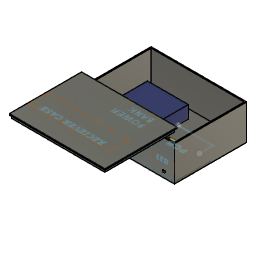
RECIEVER CASE (Autodesk Fusion 360 design; units mm, degrees)
part number: 2025-07-09-13-49-54-676
Autodesk Fusion 360 part; units mm, degrees
sketch "Sketch1" plane through (0, 0, 0) normal (0, 0, 1) x (1, 0, 0)
  line L0 (82, -62) -> (-82, -62)
  line L1 (-82, -62) -> (-82, 62)
  line L2 (-82, 62) -> (82, 62)
  line L3 (82, 62) -> (82, -62)
  line L4 (82, -62) -> (-82, 62) construction
  line L5 (-82, -62) -> (82, 62) construction
  dimension "d1" = 164
  dimension "d2" = 124
  constraint horizontal L0
  constraint perpendicular L0 L1
  constraint parallel L0 L2
  constraint parallel L1 L3
  constraint coincident L4 origin
  constraint coincident L5 origin
  measures "d1" distance of L1.end L2.end
  measures "d2" distance of L0.end L1.end
extrude "Extrude1" add sketch "Sketch1" along normal blind 60 makes body 1
shell "Shell1" thickness 2 removed faces 1 at (27.3333, -20.6667, 60) on bodies 1
sketch "Sketch2" plane through (0, 0, 0) normal (0, 0, 1) x (1, 0, 0)
  line L0 (82, -62) -> (-82, -62)
  line L1 (-82, -62) -> (-82, 62)
  line L2 (-82, 62) -> (82, 62)
  line L3 (82, 62) -> (82, -62)
  line L4 (82, -62) -> (-82, 62) construction
  line L5 (-82, -62) -> (82, 62) construction
  dimension "d6" = 164
  dimension "d7" = 124
  constraint horizontal L0
  constraint perpendicular L0 L1
  constraint parallel L0 L2
  constraint parallel L1 L3
  constraint coincident L4 origin
  constraint coincident L5 origin
  measures "d6" distance of L1.end L2.end
  measures "d7" distance of L0.end L1.end
extrude "Extrude2" add sketch "Sketch2" along normal blind 7 separate body makes body 2
move_body "Move1" bodies 2 to x (1, 0, 0) y (0, 1, 0) z (0, 0, 1) at (0, 0, 60)
sketch "Sketch3" plane through (0, 0, 67) normal (0, 0, 1) x (-1, 0, 0)
  line L0 (-82, -62) -> (82, -62)
  line L1 (82, -62) -> (82, 62)
  line L2 (82, 62) -> (-82, 62)
  line L3 (-82, 62) -> (-82, -62)
  line L4 (80, -60) -> (80, 60)
  line L5 (80, 60) -> (-80, 60)
  line L6 (-80, 60) -> (-80, -60)
  line L7 (-80, -60) -> (80, -60)
  dimension "d10" = -2
extrude "Extrude3" cut sketch "Sketch3" against normal blind 5 bodies 2
move_body "Move2" bodies 2 to x (-1, 0, 0) y (0, 1, 0) z (0, 0, -1) at (0, 0, 122)
sketch "Sketch4" plane through (0, -62, 0) normal (0, -1, 0) x (1, 0, 0)
  line L0 (-82, 0) -> (82, 0)
  line L1 (82, 0) -> (82, 60)
  line L2 (82, 60) -> (-82, 60)
  line L3 (-82, 60) -> (-82, 0)
  circle A0 centre (63.8545, 9.878) radius 2.5
  dimension "d13" = 5
  measures "d13" diameter of A0
extrude "Extrude4" cut sketch "Sketch4" against normal blind 5 contours A0 bodies 1
move_body "Move3" bodies 2 to x (1, 0, 0) y (0, 1, 0) z (0, 0, 1) at (0, 0, 30)
move_body "Move4" bodies 2 to x (1, 0, 0) y (0, 1, 0) z (0, 0, 1) at (0.6658, 0, -29.0981)
move_body "Move5" bodies 2 to x (1, 0, 0) y (0, 1, 0) z (0, 0, 1) at (0, 0, 50)
move_body "Move6" bodies 2 to x (1, 0, 0) y (0, 1, 0) z (0, 0, 1) at (0, 120, 0)
other "Base Mesh Feature1"
other "Scale1"
other "Modify1"
other "Scale2"
other "Modify2"
other "Modify3"
other "Modify4"
other "Modify5"
other "Modify6"
sketch "Sketch5" plane through (0, 0, 2) normal (0, 0, 1) x (-1, 0, 0)
  line L0 (-80, -60) -> (80, -60)
  line L1 (80, -60) -> (80, 60)
  line L2 (80, 60) -> (-80, 60)
  line L3 (-80, 60) -> (-80, -60)
  line L4 (178.7192, -8.975) -> (108.7192, -8.975)
  line L5 (108.7192, -8.975) -> (108.7192, 91.025)
  line L6 (108.7192, 91.025) -> (178.7192, 91.025)
  line L7 (178.7192, 91.025) -> (178.7192, -8.975)
  dimension "d20" = 70
  dimension "d21" = 100
  constraint horizontal L4
  constraint vertical L5
  constraint horizontal L6
  constraint vertical L7
  measures "d20" distance of L4.start L4.end
  measures "d21" distance of L4.start L6.end
extrude "Extrude5" add sketch "Sketch5" along normal blind 22 separate body contours L4 L5 L6 L7 makes body 3
move_body "Move7" bodies 3 to x (1, 0, 0) y (0, 1, 0) z (0, 0, 1) at (107.9681, 35.6096, -1.5756)
move_body "Move8" bodies 3 to x (1, 0, 0) y (0, 1, 0) z (0, 0, 1) at (0, 0, 1)
sketch "Sketch6" plane through (0, 0, 23.4244) normal (0, 0, 1) x (-1, 0, 0)
  line L0 (70.7511, 55.4154) -> (0.7511, 55.4154)
  line L1 (0.7511, 55.4154) -> (0.7511, -44.5846)
  line L2 (0.7511, -44.5846) -> (70.7511, -44.5846)
  line L3 (70.7511, -44.5846) -> (70.7511, 55.4154)
  line L4 (7.0985, -2.0355) -> (59.3473, -1.8164) construction
  line L5 (59.3473, -1.8164) -> (59.2055, 31.9775) construction
  line L6 (59.2055, 31.9775) -> (6.9568, 31.7584) construction
  line L7 (6.9568, 31.7584) -> (7.0985, -2.0355) construction
  dimension "d24" = 10
sketch "Sketch7" plane through (0, 0, 2) normal (0, 0, 1) x (-1, 0, 0)
  line L0 (-80, -60) -> (80, -60)
  line L1 (80, -60) -> (80, 60)
  line L2 (80, 60) -> (-80, 60)
  line L3 (-80, 60) -> (-80, -60)
  line L4 (-46.1522, 0) -> (-14.1367, 0) construction
  line L5 (-14.1367, 0) -> (-14.1367, 11.642) construction
  line L6 (-14.1367, 11.642) -> (-46.1522, 11.642) construction
  line L7 (-46.1522, 11.642) -> (-46.1522, 0) construction
  dimension "d25" = 10
sketch "Sketch8" plane through (0, 0, 2) normal (0, 0, 1) x (-1, 0, 0)
  line L0 (0, -26.1945) -> (-60, -26.1945)
  line L1 (-60, -26.1945) -> (-60, -2.9105)
  constraint horizontal L0
  constraint perpendicular L0 L1
move_body "Move9" bodies 2 to x (1, 0, 0) y (0, 1, 0) z (0, 0, 1) at (0, -240, -30)
other "Scale3"
sketch "Sketch9" plane through (0, 0, 82.9019) normal (0, 0, 1) x (-1, 0, 0)
  line L0 (-82.6658, 58) -> (81.3342, 58)
  line L1 (81.3342, 58) -> (81.3342, 182)
  line L2 (81.3342, 182) -> (-82.6658, 182)
  line L3 (-82.6658, 182) -> (-82.6658, 58)
sketch "Sketch10" plane through (0, -62, 0) normal (0, -1, 0) x (1, 0, 0)
  circle A0 centre (63.8545, 9.878) radius 2.5
  line L0 (-82, 0) -> (82, 0)
  line L1 (82, 0) -> (82, 60)
  line L2 (82, 60) -> (-82, 60)
  line L3 (-82, 60) -> (-82, 0)
  line L4 (40, 15.9428) -> (82, 15.9428) construction
  line L5 (82, 15.9428) -> (82, 30) construction
  line L6 (82, 30) -> (40, 30) construction
  line L7 (40, 30) -> (40, 15.9428) construction
  dimension "d30" = 8
  constraint coincident L1
sketch "Sketch11" plane through (0, 0, 2) normal (0, 0, 1) x (-1, 0, 0)
  line L0 (-60.4869, 118.2714, 80) -> (79.7623, 116.7082, 80) construction
  line L1 (79.7623, 116.7082, 80) -> (80.1246, 149.2184, 80) construction
  line L2 (80.1246, 149.2184, 80) -> (-60.1246, 150.7816, 80) construction
  line L3 (-60.1246, 150.7816, 80) -> (-60.4869, 118.2714, 80) construction
  dimension "d31" = 10
